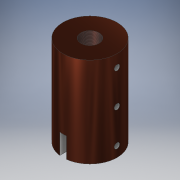
# Autodesk Inventor part: 16ghzenclosure
Saved by Autodesk Inventor 2018 (Build 220112000, 112)
## iProperties
Created: 2016-06-16
Part Number: 16ghzenclosure
Material: Generic
Document SubType Name: Modeling
Designer: Anna
Density: 1 g/cm^3
Appearance: Default
Author: Anna
Autodesk Inventor part; units mm, degrees
ref_plane "XZ Plane" through (0, 0, 0) normal (0, 1, 0) x (-1, 0, 0)
ref_plane "XY Plane" through (0, 0, 0) normal (0, 0, 1) x (1, 0, 0)
sketch "Sketch1" plane through (0, 0, 0) normal (0, 1, 0) x (-1, 0, 0)
  circle A0 centre (0, 0) radius 20
  circle A1 centre (0, 0) radius 11.05
  dimension "d0" = 40
  dimension "d1" = 22.1
  constraints: 2 centre point, 2 coincident
  measures "d0" diameter of A0
  measures "d1" diameter of A1
extrude "Extrusion1" add sketch "Sketch1" along normal blind 52.53
sketch "Sketch2" plane through (0, 0, 0) normal (0, -1, 0) x (1, 0, 0)
  circle A0 centre (0, 0) radius 13
  line L0 (0, 0) -> (9.1924, 0)
  line L1 (9.1924, 0) -> (9.1924, -9.1924)
  line L2 (9.1924, -9.1924) -> (0, -9.1924)
  line L3 (0, -9.1924) -> (0, 0)
  dimension "d4" = 26
  dimension "d5" = 9.1924
  constraints: 8 end point, 2 coincident, 2 parallel, 1 horizontal, 1 perpendicular, 3 other
  measures "d5" distance of L1.end L2.end
hole "Hole1" at (9.1924, 0, -9.1924) direction (0, 1, 0) diameter 2.2 depth 10 tip angle 118
pattern_circular "Circular Pattern1" count 4 over 360 about axis through (0, 0, 0) along (0, 1, 0) of "Hole1"
thread "Thread1" size "M2.2x0.25" class "6H" standard "ISO Metric profile" full length
thread "Thread3" size "M2.2x0.25" class "6H" standard "ISO Metric profile" full length
thread "Thread4" size "M2.2x0.25" class "6H" standard "ISO Metric profile" full length
thread "Thread5" size "M2.2x0.25" class "6H" standard "ISO Metric profile" full length
sketch "Sketch3" plane through (0, 52.53, 0) normal (0, 1, 0) x (1, 0, 0)
  circle A0 centre (0, 0) radius 20
  circle A1 centre (0, 0) radius 4.5
  dimension "d26" = 40
  dimension "d27" = 9
  constraints: 2 centre point, 2 coincident
  measures "d26" diameter of A0
  measures "d27" diameter of A1
extrude "Extrusion2" add sketch "Sketch3" along normal blind 2
sketch "Sketch4" plane through (0, 54.53, 0) normal (0, 1, 0) x (1, 0, 0)
  point P0 (0, 0)
sketch "Sketch5" plane through (0, 54.53, 0) normal (0, 1, 0) x (1, 0, 0)
  circle A0 centre (0, 0) radius 6.75
  circle A1 centre (0, 0) radius 20
  dimension "d30" = 13.5
  dimension "d31" = 40
  constraints: 2 centre point, 2 coincident
  measures "d30" diameter of A0
  measures "d31" diameter of A1
extrude "Extrusion3" add sketch "Sketch5" along normal blind 12
thread "Thread6" size "M14x0.5" class "6H" standard "ISO Metric profile" full length
sketch "Sketch8" plane through (0, 0, 0) normal (0, -1, 0) x (1, 0, 0)
  point P0 (0, 0)
sketch "Sketch9" plane through (0, 0, 0) normal (0, -1, 0) x (1, 0, 0)
  line L0 (0, 9.7277) -> (2.5, 9.7277)
  line L1 (2.5, 9.7277) -> (2.5, 16.3855)
  line L2 (2.5, 16.3855) -> (0, 16.3855)
  line L3 (0, 16.3855) -> (0, 9.7277)
  line L4 (0, 9.7277) -> (-2.5, 9.7277)
  line L5 (-2.5, 9.7277) -> (-2.5, 16.3855)
  line L6 (-2.5, 16.3855) -> (0, 16.3855)
  line L7 (0, 16.3855) -> (0, 9.7277)
  point P0 (0, 0)
  dimension "d1" = 22.1
  dimension "d54" = 2.5
  dimension "d55" = 2.5
  constraints: 16 end point, 4 parallel, 2 horizontal, 2 perpendicular, 1 point on line
  measures "d54" distance of L2.end L1.end
  measures "d55" distance of L5.end L6.end
extrude "Extrusion4" cut sketch "Sketch9" against normal blind 15
sketch "Sketch10" plane through (0, 0, 0) normal (1, 0, 0) x (0, 1, 0)
  point P0 (0, 0)
ref_plane "Work Plane1" through (20, 0, 0) normal (1, 0, 0) x (0, 1, 0)
sketch "Sketch15" plane through (0, 0, 0) normal (0, -1, 0) x (1, 0, 0)
  line L0 (2.5024, 10.6669) -> (-2.5, 10.6669)
  line L1 (-2.5, 10.6669) -> (-2.5, 24.5822)
  line L2 (-2.5, 24.5822) -> (2.5024, 24.5822)
  line L3 (2.5024, 24.5822) -> (2.5024, 10.6669)
  point P0 (0, 0)
  constraints: 8 end point, 2 parallel, 1 horizontal, 1 perpendicular
extrude "Extrusion5" cut sketch "Sketch15" against normal blind 15
sketch "Sketch18" plane through (20, 0, 0) normal (1, 0, 0) x (0, 1, 0)
  line L0 (0, 0) -> (7.575, 0)
  line L1 (7.575, 0) -> (32.575, 0)
  line L2 (32.575, 0) -> (57.575, 0)
  dimension "d102" = 7.575
  dimension "d103" = 25
  dimension "d104" = 25
  dimension "d105" = 180
  constraints: 6 end point, 3 coincident, 1 collinear, 1 horizontal, 1 point on line
  measures "d102" distance of L0.start L0.end
  measures "d103" distance of L0.end L1.end
  measures "d104" distance of L1.end L2.end
  measures "d105" angle of L2 L1
hole "Hole6" at (20, 57.575, 0) direction (-1, 0, 0) diameter 4 depth 8 tip angle 118
hole "Hole7" at (20, 7.575, 0) at (20, 32.575, 0) direction (-1, 0, 0) diameter 4 depth 8 tip angle 118
thread "Thread7" size "M4x0.7" class "6H" standard "ANSI Metric M Profile" full length
thread "Thread8" size "M4x0.7" class "6H" standard "ANSI Metric M Profile" full length
thread "Thread9" size "M4x0.7" class "6H" standard "ANSI Metric M Profile" full length
sketch "Sketch19" plane through (0, 54.53, 0) normal (0, 1, 0) x (1, 0, 0)
  circle A0 centre (0, 0) radius 6.75
  circle A1 centre (0, 0) radius 6.4
  dimension "d128" = 13.5
  dimension "d129" = 12.8
  constraints: 2 centre point, 2 coincident
  measures "d128" diameter of A0
  measures "d129" diameter of A1
extrude "Extrusion6" add sketch "Sketch19" along normal blind 2
thread "Thread11" size "M14x0.5" class "6H" standard "ANSI Metric M Profile" length 10
equation "\"d43\" = 60deg"
equation "\"Sketch6_Pitch\" = 0.5"
body "Solid1"
